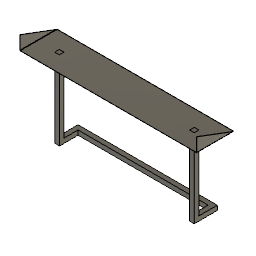
Go Kart Spoiler (Autodesk Fusion 360 design; units mm, degrees)
Autodesk Fusion 360 part; units mm, degrees
sketch "Sketch1" plane through (0, 0, 0) normal (0, 0, 1) x (1, 0, 0)
  line L0 (381, 0) -> (-381, 0)
  line L1 (-381, 0) -> (381, 0)
  line L2 (381, 0) -> (381, 25.4)
  line L3 (381, 25.4) -> (-381, 25.4)
  line L4 (-381, 25.4) -> (-381, 0)
  dimension "d1" = 762
  dimension "d2" = 25.4
  constraint midpoint L0 origin
  constraint horizontal L0
  constraint horizontal L1
  constraint vertical L2
  constraint horizontal L3
  constraint vertical L4
  measures "d1" distance of L0.start L0.end
  measures "d2" distance of L0.end L3.end
extrude "Extrude1" add sketch "Sketch1" along normal blind 25.4 makes body 1
sketch "Sketch3" plane through (0, 0, 0) normal (0, -1, 0) x (1, 0, 0)
  line L0 (-381, 0) -> (381, 0)
  line L1 (381, 0) -> (381, 25.4)
  line L2 (381, 25.4) -> (-381, 25.4)
  line L3 (-381, 25.4) -> (-381, 0)
  line L4 (-381, 25.4) -> (-355.6, 25.4)
  line L5 (-355.6, 25.4) -> (-355.6, 0)
  line L6 (-355.6, 0) -> (-381, 0)
  line L7 (-381, 0) -> (-381, 25.4)
  line L8 (381, 25.4) -> (355.6, 25.4)
  line L9 (355.6, 25.4) -> (355.6, 0)
  line L10 (355.6, 0) -> (381, 0)
  line L11 (381, 0) -> (381, 25.4)
  dimension "d7" = 25.4
  dimension "d8" = 25.4
  constraint horizontal L4
  constraint vertical L5
  constraint horizontal L6
  constraint vertical L7
  constraint coincident L2.end L3.start
  constraint horizontal L8
  constraint vertical L9
  constraint horizontal L10
  constraint vertical L11
  constraint coincident L1.end L2.start
  measures "d7" distance of L2.end L4.end
  measures "d8" distance of L1.end L8.end
extrude "Extrude2" add sketch "Sketch3" along normal blind 101.6 contours L0 L2 L3 L4 L5 L6 L7 | L0 L1 L2 L8 L9 L10 L11 bodies 1
sketch "Sketch4" plane through (0, 0, 25.4) normal (0, 0, 1) x (-1, 0, 0)
  line L0 (381, -25.4) -> (381, 101.6)
  line L1 (381, 101.6) -> (355.6, 101.6)
  line L2 (355.6, 101.6) -> (355.6, 0)
  line L3 (355.6, 0) -> (-355.6, 0)
  line L4 (-355.6, 0) -> (-355.6, 101.6)
  line L5 (-355.6, 101.6) -> (-381, 101.6)
  line L6 (-381, 101.6) -> (-381, -25.4)
  line L7 (-381, -25.4) -> (381, -25.4)
  line L8 (381, 101.6) -> (355.6, 101.6)
  line L9 (355.6, 101.6) -> (355.6, 76.2)
  line L10 (355.6, 76.2) -> (381, 76.2)
  line L11 (381, 76.2) -> (381, 101.6)
  line L12 (-355.6, 101.6) -> (-381, 101.6)
  line L13 (-381, 101.6) -> (-381, 76.2)
  line L14 (-381, 76.2) -> (-355.6, 76.2)
  line L15 (-355.6, 76.2) -> (-355.6, 101.6)
  dimension "d11" = 25.4
  dimension "d12" = 25.4
  constraint horizontal L8
  constraint vertical L9
  constraint horizontal L10
  constraint vertical L11
  constraint coincident L0.end L1.start
  constraint horizontal L12
  constraint vertical L13
  constraint horizontal L14
  constraint vertical L15
  constraint coincident L4.end L5.start
  measures "d11" distance of L0.end L10.end
  measures "d12" distance of L4.end L14.end
extrude "Extrude3" add sketch "Sketch4" along normal blind 406.4 contours L0 L1 L2 L8 L9 L10 L11 | L4 L5 L6 L12 L13 L14 L15 bodies 1
sketch "Sketch5" plane through (0, 0, 431.8) normal (0, 0, 1) x (-1, 0, 0)
  line L0 (381, 76.2) -> (381, 101.6)
  line L1 (381, 101.6) -> (355.6, 101.6)
  line L2 (355.6, 101.6) -> (355.6, 76.2)
  line L3 (355.6, 76.2) -> (381, 76.2)
  line L4 (381, 76.2) -> (381, -12.7)
  line L5 (381, 101.6) -> (381, 190.5)
  line L6 (381, 76.2) -> (381, 101.6)
  line L7 (381, 76.2) -> (381, 101.6)
  line L8 (381, -12.7) -> (-381, -12.7)
  line L9 (-381, -12.7) -> (-381, 190.5)
  line L10 (-381, 190.5) -> (381, 190.5)
  line L11 (-381, 190.5) -> (-482.6, 190.5)
  line L12 (-482.6, 190.5) -> (-482.6, -12.7)
  line L13 (-482.6, -12.7) -> (-381, -12.7)
  line L14 (-381, -12.7) -> (-381, 190.5)
  line L15 (381, 190.5) -> (482.6, 190.5)
  line L16 (482.6, 190.5) -> (482.6, -12.7)
  line L17 (482.6, -12.7) -> (381, -12.7)
  line L18 (381, -12.7) -> (381, 190.5)
  dimension "d15" = 88.9
  dimension "d16" = 88.9
  dimension "d17" = 762
  dimension "d18" = 203.2
  dimension "d27" = 203.2
  dimension "d28" = 101.6
  dimension "d29" = 101.6
  constraint coincident L0.start L3.end
  constraint perpendicular L3 L4
  constraint coincident L0.end L1.start
  constraint perpendicular L1 L5
  constraint perpendicular L4 L8
  constraint perpendicular L8 L9
  constraint horizontal L11
  constraint vertical L12
  constraint horizontal L13
  constraint vertical L14
  constraint horizontal L15
  constraint vertical L16
  constraint horizontal L17
  constraint vertical L18
  measures "d15" distance of L0.start L4.end
  measures "d16" distance of L0.end L5.end
  measures "d17" distance of L4.end L8.end
  measures "d18" distance of L8.end L9.end
  measures "d27" distance of L9.end L8.end
  measures "d28" distance of L9.end L11.end
  measures "d29" distance of L5.end L15.end
extrude "Extrude4" add sketch "Sketch5" along normal blind 1.52 separate body contours L0 L1 L2 L3 L6 L7 L18 | L1 L2 L3 L4 L5 L8 L9 L10 L14 L18 makes body 2
extrude "Extrude7" add sketch "Sketch5" along normal blind 1.52 contours L0 L4 L5 L6 L7 L15 L16 L17 L18 | L9 L11 L12 L13 L14 bodies 1 2
sketch "Sketch9" plane through (482.6, 0, 0) normal (1, 0, 0) x (0, 1, 0)
  line L0 (-190.5, 431.8) -> (12.7, 431.8)
  line L1 (12.7, 431.8) -> (12.7, 433.32)
  line L2 (12.7, 433.32) -> (-190.5, 433.32)
  line L3 (-190.5, 433.32) -> (-190.5, 431.8)
  line L4 (-190.5, 431.8) -> (12.7, 431.8)
  line L5 (-190.5, 431.8) -> (-190.5, 508)
  line L6 (-190.5, 508) -> (12.7, 431.8)
  dimension "d32" = 76.2
  constraint coincident L0.start L3.end
  constraint coincident L0.end L1.start
  constraint perpendicular L2 L5
  measures "d32" distance of L0.start L5.end
sketch "Sketch10" plane through (-482.6, 0, 0) normal (-1, 0, 0) x (0, -1, 0)
  line L0 (-12.7, 431.8) -> (190.5, 431.8)
  line L1 (190.5, 431.8) -> (190.5, 433.32)
  line L2 (190.5, 433.32) -> (-12.7, 433.32)
  line L3 (-12.7, 433.32) -> (-12.7, 431.8)
  line L4 (-12.7, 431.8) -> (190.5, 431.8)
  line L5 (190.5, 431.8) -> (190.5, 508)
  line L6 (190.5, 508) -> (-12.7, 431.8)
  dimension "d33" = 76.2
  constraint coincident L0.start L3.end
  constraint coincident L0.end L1.start
  constraint perpendicular L0 L5
  measures "d33" distance of L0.end L5.end
extrude "Extrude8" add sketch "Sketch9" along normal blind 1.52 separate body contours L2 L5 L6 makes body 3
extrude "Extrude9" add sketch "Sketch10" along normal blind 1.52 separate body contours L2 L5 L6 makes body 4
